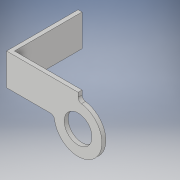
# Autodesk Inventor part: Pivot Bracket Other Side
Saved by Autodesk Inventor 2017 (Build 210142000, 142)
## iProperties
Created: 2017-06-10
Part Number: Pivot Bracket Other Side
Material: Generic
Document SubType Name: Modeling
Designer: Matthew
Density: 1 g/cm^3
Appearance: Default
Author: Matthew
Autodesk Inventor part; units mm, degrees
ref_plane "YZ Plane" through (0, 0, 0) normal (1, 0, 0) x (0, 1, 0)
ref_plane "XZ Plane" through (0, 0, 0) normal (0, 1, 0) x (-1, 0, 0)
ref_plane "XY Plane" through (0, 0, 0) normal (0, 0, 1) x (1, 0, 0)
sketch "Sketch1" plane through (0, 0, 0) normal (0, 1, 0) x (-1, 0, 0)
  line L0 (0, 0) -> (57.15, 0)
  line L1 (112.534, 31.2241) -> (58.0687, -3.175)
  line L2 (58.0687, -3.175) -> (0, -3.175)
  line L3 (0, -3.175) -> (0, 0)
  line L4 (110.8385, 33.9086) -> (112.534, 31.2241)
  line L5 (57.15, 0) -> (110.8385, 33.9086)
  dimension "d0" = 3.175
  dimension "d1" = 3.175
  dimension "d3" = 57.15
  dimension "d4" = 63.5
  dimension "d5" = 147.724
  constraints: 12 end point, 2 parallel, 2 perpendicular, 1 horizontal
  measures "d0" distance of L2.end L0.start
  measures "d1" distance of L4.start L1.start
  measures "d3" distance of L0.start L0.end
  measures "d4" distance of L0.end L4.start
  measures "d5" angle of L0 L5
extrude "Extrusion1" add sketch "Sketch1" along normal blind 25.4
sketch "Sketch4" plane through (-57.15, 0, 0) normal (0, 0, 1) x (1, 0, 0)
  circle A0 centre (57.15, 0) radius 19.05
  dimension "d15" = 38.1
  constraints: 1 centre point, 1 coincident
  measures "d15" diameter of A0
extrude "Extrusion4" add sketch "Sketch4" against normal blind 3.175
sketch "Sketch5" plane through (-57.15, 25.4, 0) normal (0, 0, 1) x (1, 0, 0)
  circle A0 centre (57.15, -25.4) radius 11.1125
  dimension "d18" = 22.225
  constraints: 1 centre point, 1 coincident
  measures "d18" diameter of A0
extrude "Extrusion5" cut sketch "Sketch5" against normal blind 3.175
fillet "Fillet2" radius 3.175 2 edges at (0, 19.05, -1.5875) (-19.05, 0, -1.5875)
sketch "Sketch6" plane through (0, 25.4, 0) normal (0, 1, 0) x (1, 0, 0)
  line L0 (-57.15, 0) -> (0, 0) projected
  line L1 (0, 0) -> (-57.15, 0)
  line L2 (-135.8522, 42.4181) -> (-57.15, 42.4181)
  line L3 (-57.15, 42.4181) -> (-57.15, -51.2232)
  line L4 (-57.15, -51.2232) -> (-135.8522, -51.2232)
  line L5 (-135.8522, -51.2232) -> (-135.8522, 42.4181)
  dimension "d22" = 57.15
  constraints: 10 end point, 2 horizontal, 2 parallel, 1 perpendicular
  measures "d22" distance of L0.end L0.start
extrude "Extrusion6" cut sketch "Sketch6" against normal blind 61.9125
sketch "Sketch7" plane through (0, 25.4, 0) normal (0, 1, 0) x (1, 0, 0)
  line L0 (-57.15, 0) -> (0, 0) projected
  line L1 (0, 0) -> (-57.15, 0)
  line L2 (-57.15, 0) -> (-53.975, 0)
  line L3 (-53.975, 0) -> (-53.975, 57.15)
  line L4 (-53.975, 57.15) -> (-57.15, 57.15)
  line L5 (-57.15, 57.15) -> (-57.15, 0)
  dimension "d25" = 57.15
  dimension "d26" = 3.175
  dimension "d27" = 57.15
  constraints: 10 end point, 2 horizontal, 2 parallel, 1 perpendicular
  measures "d25" distance of L0.end L0.start
  measures "d26" distance of L4.end L3.end
  measures "d27" distance of L3.end L2.end
extrude "Extrusion7" add sketch "Sketch7" against normal up to surface (25.4 mm away)
body "Solid1"
